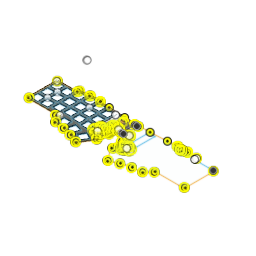
chillboardassembly (Autodesk Fusion 360 archive; units mm, degrees)
design "chillboardplate"
Autodesk Fusion 360 part; units mm, degrees
sketch "Sketch1" plane through (0, 0, 1.51) normal (0, 0, 1) x (-1, 0, 0)
  arc A0 (-249.2993, 48.4492) -> (-248.7993, 47.9492) centre (-248.7995, 48.449) ccw
  line L0 (-248.7993, 47.9492) -> (-230.2493, 47.9511)
  arc A1 (-230.2493, 47.9511) -> (-229.8152, 48.3951) centre (-230.2593, 48.3951) ccw
  line L1 (-229.8152, 48.3951) -> (-229.8152, 49.6471)
  arc A2 (-229.3152, 50.1471) -> (-229.8152, 49.6471) centre (-229.3152, 49.6471) ccw
  line L2 (-229.3152, 50.1471) -> (-211.372, 50.1471)
  line L3 (-211.372, 50.1471) -> (-211.2585, 50.1504)
  line L4 (-211.2585, 50.1504) -> (-179.6466, 51.9479)
  line L5 (-179.6466, 51.9479) -> (-179.5319, 51.9511)
  line L6 (-179.5319, 51.9511) -> (-158.6013, 51.939)
  arc A3 (-158.6013, 51.939) -> (-156.6002, 53.9398) centre (-158.6, 53.9389) ccw
  line L7 (-156.6002, 53.9398) -> (-156.6033, 54.58)
  line L8 (-153.5416, 54.58) -> (-153.5408, 54.0387)
  arc A4 (-153.5408, 54.0387) -> (-151.5397, 52.0379) centre (-151.5408, 54.0379) ccw
  line L9 (-151.5397, 52.0379) -> (-130.609, 52.05)
  line L10 (-130.609, 52.05) -> (-130.4943, 52.0467)
  line L11 (-130.4943, 52.0467) -> (-98.8825, 50.2492)
  line L12 (-98.8825, 50.2492) -> (-98.7689, 50.246)
  line L13 (-98.7689, 50.246) -> (-80.8258, 50.246)
  arc A5 (-80.3258, 49.746) -> (-80.8258, 50.246) centre (-80.8257, 49.746) ccw
  line L14 (-80.3258, 49.746) -> (-80.3258, 48.494)
  arc A6 (-80.3258, 48.494) -> (-79.8916, 48.05) centre (-79.8816, 48.494) ccw
  line L15 (-79.8916, 48.05) -> (-61.3416, 48.048)
  arc A7 (-61.3416, 48.048) -> (-60.8416, 48.548) centre (-61.3416, 48.548) ccw
  line L16 (-60.8416, 48.548) -> (-60.8416, 49.8)
  arc A8 (-60.3416, 50.3) -> (-60.8416, 49.8) centre (-60.3416, 49.8) ccw
  line L17 (-60.3416, 50.3) -> (-42.3416, 50.3)
  arc A9 (-42.3416, 50.3) -> (-41.8416, 50.8) centre (-42.3416, 50.8) ccw
  line L18 (-41.8416, 50.8) -> (-41.8416, 54.549)
  arc A10 (-41.3416, 55.049) -> (-41.8416, 54.549) centre (-41.3416, 54.549) ccw
  line L19 (-41.3416, 55.049) -> (-5.221, 55.0499)
  line L20 (-5.221, 55.0499) -> (-4.241, 55.0499)
  arc A11 (-4.241, 55.0499) -> (-3.241, 56.0493) centre (-4.241, 56.05) ccw
  line L21 (-3.241, 56.0493) -> (-3.206, 111.2252)
  arc A12 (-3.206, 111.2252) -> (-5.2063, 113.2259) centre (-5.206, 111.2259) ccw
  line L22 (-5.2063, 113.2259) -> (-59.5413, 113.2163)
  arc A13 (-61.2133, 114.1182) -> (-59.5413, 113.2163) centre (-59.5417, 115.2163) ccw
  line L23 (-61.2133, 114.1182) -> (-69.6969, 126.8008)
  arc A14 (-69.6969, 126.8008) -> (-71.3614, 127.6889) centre (-71.3592, 125.6889) ccw
  line L24 (-71.3614, 127.6889) -> (-89.0903, 127.67)
  arc A15 (-89.6042, 127.7371) -> (-89.0903, 127.67) centre (-89.0903, 129.67) ccw
  line L25 (-89.6042, 127.7371) -> (-107.2475, 132.428)
  arc A16 (-107.7624, 132.6457) -> (-107.2475, 132.428) centre (-106.7336, 134.3608) ccw
  line L26 (-107.7624, 132.6457) -> (-122.862, 141.7034)
  arc A17 (-122.862, 141.7034) -> (-125.6008, 140.9797) centre (-123.8706, 139.9763) ccw
  line L27 (-125.6008, 140.9797) -> (-140.9575, 115.8859)
  arc A18 (-140.9575, 115.8859) -> (-141.2516, 114.8416) centre (-139.2515, 114.8419) ccw
  line L28 (-141.2515, 114.8416) -> (-141.2485, 95.035)
  arc A19 (-141.8356, 93.6196) -> (-141.2485, 95.035) centre (-143.2486, 95.0352) ccw
  line L29 (-141.8356, 93.6196) -> (-152.9976, 82.4783)
  arc A20 (-152.9976, 82.4783) -> (-153.5297, 81.1213) centre (-151.5299, 81.1199) ccw
  line L30 (-153.5297, 81.1213) -> (-153.53, 80.46)
  line L31 (-156.5941, 80.46) -> (-156.6113, 81.0225)
  arc A21 (-156.6113, 81.0225) -> (-157.1434, 82.3794) centre (-158.6116, 81.0209) ccw
  line L32 (-157.1434, 82.3794) -> (-168.3054, 93.5208)
  arc A22 (-168.8925, 94.9362) -> (-168.3054, 93.5208) centre (-166.8921, 94.9365) ccw
  line L33 (-168.8925, 94.9362) -> (-168.8894, 114.7428)
  arc A23 (-168.8894, 114.7428) -> (-169.1835, 115.787) centre (-170.8895, 114.7431) ccw
  line L34 (-169.1835, 115.787) -> (-184.5401, 140.8808)
  arc A24 (-184.5401, 140.8808) -> (-187.279, 141.6046) centre (-186.2703, 139.8775) ccw
  line L35 (-187.279, 141.6046) -> (-202.3786, 132.5469)
  arc A25 (-202.8935, 132.3291) -> (-202.3786, 132.5469) centre (-203.4077, 134.2626) ccw
  line L36 (-202.8935, 132.3291) -> (-220.5368, 127.6383)
  arc A26 (-221.0507, 127.5711) -> (-220.5368, 127.6383) centre (-221.0505, 129.5701) ccw
  line L37 (-221.0507, 127.5711) -> (-238.7796, 127.59)
  arc A27 (-238.7796, 127.59) -> (-240.4441, 126.702) centre (-238.7818, 125.5901) ccw
  line L38 (-240.4441, 126.702) -> (-248.9277, 114.0194)
  arc A28 (-250.5997, 113.1174) -> (-248.9277, 114.0194) centre (-250.5993, 115.1174) ccw
  line L39 (-250.5997, 113.1174) -> (-304.9347, 113.1271)
  arc A29 (-304.9347, 113.1271) -> (-306.935, 111.1264) centre (-304.935, 111.1271) ccw
  line L40 (-306.935, 111.1264) -> (-306.9, 55.9505)
  arc A30 (-306.9, 55.9505) -> (-305.9, 54.9511) centre (-305.8999, 55.9512) ccw
  line L41 (-305.9, 54.9511) -> (-304.92, 54.9511)
  arc A31 (-268.2993, 50.7012) -> (-267.7993, 50.2012) centre (-267.7995, 50.701) ccw
  line L42 (-267.7993, 50.2012) -> (-249.7993, 50.2012)
  arc A32 (-249.2993, 49.7012) -> (-249.7993, 50.2012) centre (-249.7995, 49.701) ccw
  line L43 (-249.2993, 49.7012) -> (-249.2993, 48.4492)
  circle A33 centre (-138.351, 114.92) radius 0.4
  arc A34 (-127.6766, 107.43) -> (-127.6766, 105.93) centre (-127.6766, 106.68) ccw
  line L44 (-127.6766, 107.43) -> (-126.3766, 107.43)
  arc A35 (-126.3766, 105.93) -> (-126.3766, 107.43) centre (-126.3766, 106.68) ccw
  line L45 (-126.3766, 105.93) -> (-127.6766, 105.93)
  circle A36 centre (-136.8516, 106.16) radius 0.4
  circle A37 centre (-119.5266, 103.58) radius 0.5
  circle A38 centre (-134.0266, 103.58) radius 0.5
  circle A39 centre (-119.5266, 101.08) radius 0.5
  circle A40 centre (-119.5266, 98.58) radius 0.5
  circle A41 centre (-134.0266, 98.58) radius 0.5
  circle A42 centre (-136.8516, 96) radius 0.4
  arc A43 (-127.6766, 96.23) -> (-127.6766, 94.73) centre (-127.6766, 95.48) ccw
  line L46 (-127.6766, 96.23) -> (-126.3766, 96.23)
  arc A44 (-126.3766, 94.73) -> (-126.3766, 96.23) centre (-126.3766, 95.48) ccw
  line L47 (-126.3766, 94.73) -> (-127.6766, 94.73)
  circle A45 centre (-131.9516, 92.48) radius 0.4
  circle A46 centre (-139.5716, 92.48) radius 0.4
  circle A47 centre (-173.5116, 106.03) radius 0.4
  circle A48 centre (-180.811, 109.71) radius 0.4
  arc A49 (-184.7752, 107.9098) -> (-184.7752, 106.4098) centre (-184.7752, 107.1598) ccw
  line L48 (-184.7752, 107.9098) -> (-183.4752, 107.9098)
  arc A50 (-183.4752, 106.4098) -> (-183.4752, 107.9098) centre (-183.4752, 107.1598) ccw
  line L49 (-183.4752, 106.4098) -> (-184.7752, 106.4098)
  circle A51 centre (-176.6252, 104.0598) radius 0.5
  circle A52 centre (-191.1252, 104.0598) radius 0.5
  circle A53 centre (-176.6252, 101.5598) radius 0.5
  circle A54 centre (-173.5116, 95.87) radius 0.4
  circle A55 centre (-176.6252, 99.0598) radius 0.5
  circle A56 centre (-191.1252, 99.0598) radius 0.5
  arc A57 (-184.7752, 96.7098) -> (-184.7752, 95.2098) centre (-184.7752, 95.9598) ccw
  line L50 (-184.7752, 96.7098) -> (-183.4752, 96.7098)
  arc A58 (-183.4752, 95.2098) -> (-183.4752, 96.7098) centre (-183.4752, 95.9598) ccw
  line L51 (-183.4752, 95.2098) -> (-184.7752, 95.2098)
  circle A59 centre (-120.9266, 89.795) radius 0.5
  circle A60 centre (-123.4666, 89.795) radius 0.5
  circle A61 centre (-126.0066, 89.795) radius 0.5
  circle A62 centre (-128.5466, 89.795) radius 0.5
  circle A63 centre (-131.9516, 89.94) radius 0.4
  circle A64 centre (-131.9516, 87.4) radius 0.4
  circle A65 centre (-139.5716, 89.94) radius 0.4
  circle A66 centre (-139.5716, 87.4) radius 0.4
  circle A67 centre (-131.9516, 84.86) radius 0.4
  circle A68 centre (-131.9516, 82.32) radius 0.4
  circle A69 centre (-139.5716, 84.86) radius 0.4
  circle A70 centre (-139.5716, 82.32) radius 0.4
  circle A71 centre (-131.9516, 79.78) radius 0.4
  circle A72 centre (-131.9516, 77.24) radius 0.4
  circle A73 centre (-139.5716, 79.78) radius 0.4
  circle A74 centre (-145.0516, 80.62) radius 0.325
  circle A75 centre (-139.5716, 77.24) radius 0.4
  circle A76 centre (-142.5116, 78.08) radius 0.325
  circle A77 centre (-147.5916, 78.08) radius 0.325
  circle A78 centre (-131.9516, 74.7) radius 0.4
  circle A79 centre (-145.0516, 75.54) radius 0.325
  circle A80 centre (-139.5716, 74.7) radius 0.4
  circle A81 centre (-136.1516, 63.08) radius 1.25
  circle A82 centre (-136.1516, 59.68) radius 1.25
  circle A83 centre (-165.3116, 80.49) radius 0.325
  circle A84 centre (-162.7716, 77.95) radius 0.325
  circle A85 centre (-167.8516, 77.95) radius 0.325
  circle A86 centre (-165.3116, 75.41) radius 0.325
  arc A87 (-238.5649, 51.3817) -> (-237.8622, 52.0303) centre (-238.3127, 51.8134) ccw
  arc A88 (-238.5649, 51.3817) -> (-238.8172, 51.45) centre (-238.8172, 50.95) ccw
  line L52 (-238.8172, 51.45) -> (-240.4061, 51.45)
  arc A89 (-240.4061, 51.45) -> (-240.6583, 51.3817) centre (-240.4061, 50.95) ccw
  arc A90 (-241.3611, 52.0303) -> (-240.6583, 51.3817) centre (-240.9106, 51.8134) ccw
  arc A91 (-241.3611, 52.0303) -> (-241.3116, 52.2472) centre (-241.812, 52.2472) ccw
  arc A92 (-237.9116, 52.2472) -> (-237.8622, 52.0303) centre (-237.4116, 52.2472) ccw
  line L53 (-153.5416, 54.58) -> (-153.53, 80.46)
  line L54 (-156.6033, 54.58) -> (-156.5941, 80.46)
  arc A93 (-268.2993, 54.4502) -> (-268.7991, 54.9504) centre (-268.7994, 54.4504) ccw
  line L55 (-268.2993, 50.7012) -> (-268.2993, 54.4502)
  line L56 (-304.92, 54.9511) -> (-268.7991, 54.9504)
  line L57 (-179.3299, 92.4458) -> (-191.3299, 92.4458)
  line L58 (-191.3299, 92.4458) -> (-191.3299, 54.4458)
  line L59 (-191.3299, 54.4458) -> (-179.3299, 54.4458)
  line L60 (-179.3299, 54.4458) -> (-179.3299, 92.4458)
  circle A94 centre (-165.3116, 77.95) radius 4.55
  circle A95 centre (-184.1252, 101.5598) radius 3
  line L61 (-118.7366, 90.8515) -> (-130.7366, 90.8515)
  line L62 (-130.7366, 90.8515) -> (-130.7366, 52.8515)
  line L63 (-130.7366, 52.8515) -> (-118.7366, 52.8515)
  line L64 (-118.7366, 52.8515) -> (-118.7366, 90.8515)
  arc A96 (-3.9437, 56.1615) -> (-4.4437, 56.6615) centre (-3.9437, 56.6615) cw
  line L65 (-77.2641, 51.1516) -> (-63.4641, 51.1507)
  line L66 (-58.2639, 53.5253) -> (-44.4639, 53.5243)
  line L67 (-39.2609, 96.2739) -> (-25.4609, 96.273)
  line L68 (-44.4602, 105.3243) -> (-58.2602, 105.3253)
  line L69 (-6.4599, 110.0716) -> (-20.2599, 110.0726)
  line L70 (-77.2627, 70.1516) -> (-63.4627, 70.1507)
  line L71 (-77.2617, 83.9516) -> (-77.2627, 70.1516)
  line L72 (-44.4639, 53.5243) -> (-44.4629, 67.3243)
  line L73 (-63.4617, 83.9507) -> (-77.2617, 83.9516)
  line L74 (-101.461, 93.9034) -> (-101.46, 107.7034)
  line L75 (-6.4622, 77.2716) -> (-6.4612, 91.0716)
  line L76 (-6.4626, 72.0716) -> (-20.2626, 72.0726)
  line L77 (-77.2604, 102.9516) -> (-77.2614, 89.1516)
  line L78 (-96.2602, 105.328) -> (-96.2612, 91.528)
  line L79 (-58.2612, 91.5253) -> (-44.4612, 91.5243)
  line L80 (-82.4625, 72.527) -> (-82.4616, 86.327)
  line L81 (-20.2612, 91.0726) -> (-20.2622, 77.2726)
  line L82 (-20.2636, 58.2726) -> (-6.4636, 58.2716)
  line L83 (-20.2609, 96.2726) -> (-6.4609, 96.2716)
  line L84 (-39.2636, 58.2739) -> (-25.4636, 58.273)
  line L85 (-58.2602, 105.3253) -> (-58.2612, 91.5253)
  line L86 (-6.4636, 58.2716) -> (-6.4626, 72.0716)
  line L87 (-82.4612, 91.527) -> (-82.4602, 105.327)
  line L88 (-96.2625, 72.528) -> (-82.4625, 72.527)
  line L89 (-72.9598, 111.1513) -> (-72.9588, 124.9513)
  line L90 (-44.4612, 91.5243) -> (-44.4602, 105.3243)
  line L91 (-115.261, 93.9044) -> (-101.461, 93.9034)
  line L92 (-44.4625, 72.5243) -> (-44.4616, 86.3243)
  line L93 (-44.4616, 86.3243) -> (-58.2616, 86.3253)
  line L94 (-20.2622, 77.2726) -> (-6.4622, 77.2716)
  line L95 (-82.4602, 105.327) -> (-96.2602, 105.328)
  line L96 (-109.5034, 115.9767) -> (-95.9807, 112.3522)
  line L97 (-95.9807, 112.3522) -> (-92.3563, 125.8749)
  line L98 (-92.3563, 125.8749) -> (-105.879, 129.4994)
  line L99 (-96.2612, 91.528) -> (-82.4612, 91.527)
  line L100 (-44.4629, 67.3243) -> (-58.2629, 67.3253)
  line L101 (-82.4639, 53.527) -> (-82.4629, 67.327)
  line L102 (-82.4616, 86.327) -> (-96.2616, 86.328)
  line L103 (-86.7588, 124.9523) -> (-86.7598, 111.1523)
  line L104 (-101.46, 107.7034) -> (-115.26, 107.7044)
  arc A97 (-117.4706, 56.4267) -> (-117.4706, 56.4269) centre (-116.9706, 56.4268) cw
  line L105 (-105.879, 129.4994) -> (-109.5034, 115.9767)
  line L106 (-101.4624, 74.9034) -> (-101.4614, 88.7034)
  line L107 (-86.7598, 111.1523) -> (-72.9598, 111.1513)
  line L108 (-58.2616, 86.3253) -> (-58.2625, 72.5253)
  line L109 (-77.2631, 64.9516) -> (-77.2641, 51.1516)
  line L110 (-96.2629, 67.328) -> (-96.2639, 53.528)
  line L111 (-96.2616, 86.328) -> (-96.2625, 72.528)
  line L112 (-63.4631, 64.9507) -> (-77.2631, 64.9516)
  line L113 (-63.4604, 102.9507) -> (-77.2604, 102.9516)
  line L114 (-115.2637, 55.9044) -> (-101.4637, 55.9034)
  line L115 (-63.4641, 51.1507) -> (-63.4631, 64.9507)
  line L116 (-63.4627, 70.1507) -> (-63.4617, 83.9507)
  line L117 (-72.9588, 124.9513) -> (-86.7588, 124.9523)
  line L118 (-101.4637, 55.9034) -> (-101.4627, 69.7034)
  line L119 (-115.26, 107.7044) -> (-115.261, 93.9044)
  line L120 (-115.2624, 74.9044) -> (-101.4624, 74.9034)
  line L121 (-101.4614, 88.7034) -> (-115.2614, 88.7044)
  line L122 (-77.2614, 89.1516) -> (-63.4614, 89.1507)
  line L123 (-115.2614, 88.7044) -> (-115.2624, 74.9044)
  line L124 (-82.4629, 67.327) -> (-96.2629, 67.328)
  line L125 (-101.4627, 69.7034) -> (-115.2627, 69.7044)
  line L126 (-96.2639, 53.528) -> (-82.4639, 53.527)
  line L127 (-58.2625, 72.5253) -> (-44.4625, 72.5243)
  line L128 (-39.2612, 91.0739) -> (-39.2622, 77.2739)
  line L129 (-63.4614, 89.1507) -> (-63.4604, 102.9507)
  line L130 (-115.2627, 69.7044) -> (-115.2637, 55.9044)
  line L131 (-39.2622, 77.2739) -> (-25.4622, 77.273)
  line L132 (-25.4622, 77.273) -> (-25.4612, 91.073)
  line L133 (-39.2599, 110.0739) -> (-39.2609, 96.2739)
  line L134 (-20.2626, 72.0726) -> (-20.2636, 58.2726)
  line L135 (-39.2626, 72.0739) -> (-39.2636, 58.2739)
  line L136 (-25.4612, 91.073) -> (-39.2612, 91.0739)
  line L137 (-25.4636, 58.273) -> (-25.4626, 72.073)
  line L138 (-6.4609, 96.2716) -> (-6.4599, 110.0716)
  line L139 (-20.2599, 110.0726) -> (-20.2609, 96.2726)
  line L140 (-25.4609, 96.273) -> (-25.4599, 110.073)
  line L141 (-25.4626, 72.073) -> (-39.2626, 72.0739)
  line L142 (-25.4599, 110.073) -> (-39.2599, 110.0739)
  line L143 (-6.4612, 91.0716) -> (-20.2612, 91.0726)
  line L144 (-58.2629, 67.3253) -> (-58.2639, 53.5253)
  circle A98 centre (-127.0266, 101.08) radius 4.5
  circle A99 centre (-22.9514, 74.4045) radius 2
  circle A100 centre (-22.9514, 93.4595) radius 2
  circle A101 centre (-64.2322, 110.9003) radius 2
  circle A102 centre (-79.9323, 69.705) radius 2
  line L145 (-125.6648, 133.9038) -> (-113.541, 126.903)
  line L146 (-132.6657, 121.78) -> (-120.5418, 114.7791)
  line L147 (-125.6648, 133.9038) -> (-132.6657, 121.78)
  line L148 (-120.5418, 114.7791) -> (-113.541, 126.903)
  circle A103 centre (-145.0516, 78.0808) radius 5
  point P0 (3.4618, -8.3499)
  point P1 (1.4614, -6.3492)
  point P2 (1.4618, -8.3492)
  dimension "d6" = 12
  dimension "d9" = 9.1
  dimension "d10" = 6
  dimension "d13" = 7.5
  dimension "d15" = 12
  dimension "d16" = 38
  dimension "d18" = 4
  dimension "d19" = 19.722
  dimension "d20" = 4
  dimension "d21" = 19.055
  dimension "d22" = 19.355
  dimension "d23" = 4
  dimension "d24" = 61.026
  dimension "d25" = 62.852
  dimension "d26" = 4
  dimension "d27" = 76.7
  dimension "d33" = 14
  dimension "d35" = 14
  dimension "d36" = 14
  dimension "d37" = 14
  dimension "d38" = 14
  dimension "d39" = 0.014
  dimension "d40" = 2.19
  dimension "d43" = 21.655
  dimension "d46" = 9
  dimension "d47" = 10
  constraint coincident L8.start L53.start
  constraint coincident L30.end L53.end
  constraint coincident L7.end L54.start
  constraint coincident L31.start L54.end
  constraint coincident L41.end L56.start
  constraint horizontal L57
  constraint vertical L58
  constraint horizontal L59
  constraint vertical L60
  constraint collinear A84.centre A85.centre A94.centre
  constraint collinear A83.centre A86.centre A94.centre
  constraint horizontal A53.centre A95.centre
  constraint horizontal L61
  constraint vertical L62
  constraint horizontal L63
  constraint horizontal A39.centre A98.centre
  constraint vertical A99.centre A100.centre
  constraint perpendicular L146 L147
  constraint perpendicular L145 L148
  constraint collinear A74.centre A79.centre A103.centre
  measures "d6" distance of L58 L60
  measures "d9" diameter of A94
  measures "d10" diameter of A95
  measures "d13" horizontal distance of A53.centre A95.centre
  measures "d15" distance of L62 L64
  measures "d16" distance of L61 L63
  measures "d18" diameter of A99
  measures "d19" distance of L21 A99.centre
  measures "d20" diameter of A100
  measures "d21" vertical distance of A99.centre A100.centre
  measures "d22" distance of L19 A99.centre
  measures "d23" diameter of A101
  measures "d24" distance of L21 A101.centre
  measures "d25" distance of L15 A101.centre
  measures "d26" diameter of A102
  measures "d27" distance of L21 A102.centre
  measures "d33" distance of L145.start L145.end
  measures "d35" distance of L146.start L146.end
  measures "d36" distance of L145.start L146.start
  measures "d37" distance of L97 L105
  measures "d38" distance of L96 L98
  measures "d39" angle of L22 L69
  measures "d40" distance of A62.centre L62
  measures "d43" distance of L15 A102.centre
  measures "d46" diameter of A98
  measures "d47" diameter of A103
extrude "Extrude2" add sketch "Sketch1" along normal blind 1.2 contours L8 A4 L9 L10 L11 L12 L13 A5 L14 A6 L15 A7 L16 A8 L17 A9 L18 A10 L19 L20 A11 L21 A12 L22 A13 L23 A14 L24 A15 L25 A16 L26 A17 L27 A18 L28 A19 L29 A20 L30 L53 | A33 | A36 | A37 | A38 | A39 | A40 | A41 | A42 | A45 | A63 | A64 | A65 | A66 | A67 | A68 | A69 | A70 | A71 | A72 | A73 | A75 | A78 | A80 | A81 | A82 | A97
extrude "Extrude3" add sketch "Sketch1" along normal blind 1.2 contours A34 L44 A35 L45 | A43 L46 A44 L47
extrude "Extrude1" [suppressed]
